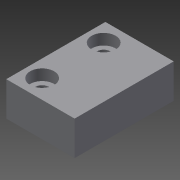
# Autodesk Inventor part: YIdlerCapLeft
Saved by Autodesk Inventor 2015 (Build 190159000, 159)
## iProperties
Created: 2014-08-15
Part Number: YIdlerCapLeft
Material: Generic
Document SubType Name: Modeling
Designer: t_clevj
Density: 1 g/cm^3
Appearance: Default
Author: t_clevj
Autodesk Inventor part; units mm, degrees
ref_plane "YZ Plane" through (0, 0, 0) normal (1, 0, 0) x (0, 1, 0)
ref_plane "XZ Plane" through (0, 0, 0) normal (0, 1, 0) x (-1, 0, 0)
ref_plane "XY Plane" through (0, 0, 0) normal (0, 0, 1) x (1, 0, 0)
sketch "Sketch1" plane through (0, 0, 0) normal (0, 0, 1) x (1, 0, 0)
  line L0 (0, 0) -> (20, 0)
  line L1 (20, 0) -> (20, 29)
  line L2 (20, 29) -> (0, 29)
  line L3 (0, 29) -> (0, 0)
  dimension "d0" = 29
  dimension "d1" = 20
  constraints: 8 end point, 2 parallel, 1 horizontal, 1 perpendicular
  measures "d0" distance of L2.end L0.start
  measures "d1" distance of L0.start L0.end
extrude "Extrusion1" add sketch "Sketch1" along normal blind 10
sketch "Sketch2" plane through (0, 0, 10) normal (0, 0, 1) x (1, 0, 0)
  line L0 (0, 0) -> (20, 0) projected
  line L1 (0, 29) -> (0, 0) projected
  point P0 (5, 23.5)
  point P1 (5, 5.5)
  dimension "d4" = 5.5
  dimension "d5" = 5
  dimension "d6" = 23.5
  constraints: 1 vertical alignment
  measures "d4" distance from line of L0 point (5, 5.5)
  measures "d5" distance from line of L1 point (5, 5.5)
  measures "d6" distance from line of L0 point (5, 23.5)
hole "Hole1" at (5, 23.5, 10) at (5, 5.5, 10) direction (0, 0, -1) diameter 4 end up to face face through (6.6667, 19.3333, 0) facing (0, 0, -1) counterbore diameter 7 counterbore depth 3.2
body "Solid1"
